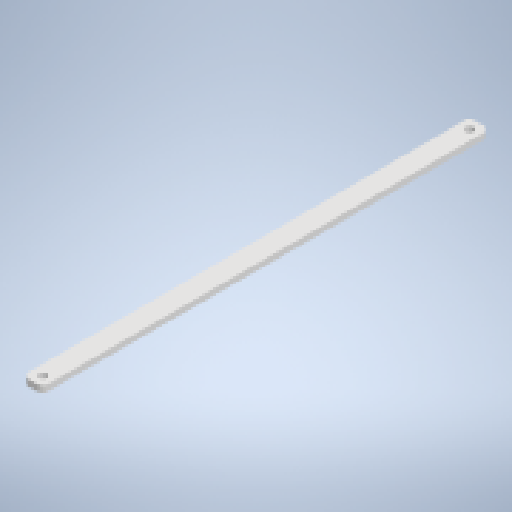
# Autodesk Inventor part: Tensor
Saved by Autodesk Inventor 2024 (Build 280153000, 153)
## iProperties
Created: 2025-02-23
Part Number: Tensor
Material: Genérico
Document SubType Name: Modeling
Designer: sergi
Density: 1 g/cm^3
Appearance: Valor por defecto
Author: sergi
Autodesk Inventor part; units mm, degrees
ref_plane "YZ Plane" through (0, 0, 0) normal (1, 0, 0) x (0, 1, 0)
ref_plane "XZ Plane" through (0, 0, 0) normal (0, 1, 0) x (-1, 0, 0)
ref_plane "XY Plane" through (0, 0, 0) normal (0, 0, 1) x (1, 0, 0)
sketch "Boceto1" plane through (0, 0, 0) normal (0, 1, 0) x (-1, 0, 0)
  line L0 (-2, 110) -> (2, 110)
  line L1 (5, 107) -> (5, -107)
  line L2 (2, -110) -> (-2, -110)
  line L3 (-5, -107) -> (-5, 107)
  line L4 (-5, 110) -> (5, -110) construction
  line L5 (5, 110) -> (-5, -110) construction
  arc A0 (5, 107) -> (2, 110) centre (2, 107) ccw
  arc A1 (-2, 110) -> (-5, 107) centre (-2, 107) ccw
  arc A2 (-5, -107) -> (-2, -110) centre (-2, -107) ccw
  arc A3 (2, -110) -> (5, -107) centre (2, -107) ccw
  point P0 (0, 0)
  dimension "d0" = 10
  dimension "d1" = 220
  dimension "d2" = 3
  constraints: 12 end point, 8 point on circle, 8 point on line, 8 tangent, 4 centre point, 3 equal radius, 2 midpoint, 2 parallel, 1 horizontal, 1 perpendicular
  measures "d0" distance of L4.end L5.end
  measures "d1" distance of L5.start L4.end
  measures "d2" radius of A0
extrude "Extrusión1" add sketch "Boceto1" along normal blind 3
sketch "Boceto2" plane through (0, 3, 0) normal (0, 1, 0) x (1, 0, 0)
  line L0 (5, -107) -> (5, 107) projected
  line L1 (-2, -110) -> (2, -110) projected
  line L2 (2, 110) -> (-2, 110) projected
  point P0 (0, 0)
  point P1 (0, -105)
  point P2 (0, 105)
  dimension "d5" = 5
  dimension "d6" = 5
  dimension "d7" = 5
  dimension "d8" = 5
  measures "d5" distance from line of L0 point (0, -105)
  measures "d6" distance from line of L1 point (0, -105)
  measures "d7" distance from line of L2 point (0, 105)
  measures "d8" distance from line of L0 point (0, 105)
hole "Agujero1" at (0, 3, 105) at (0, 3, -105) direction (0, -1, 0) diameter 4.2 end through all
